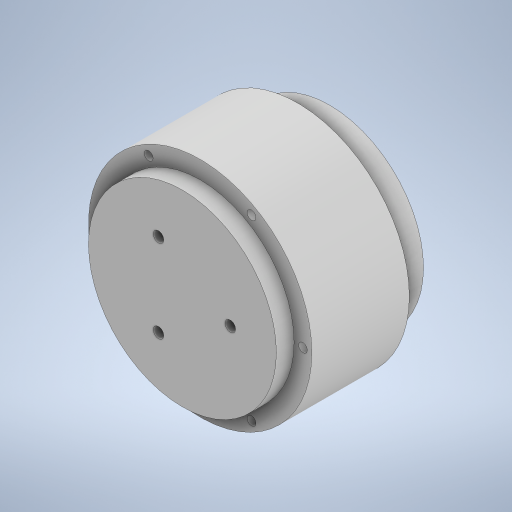
# Autodesk Inventor part: 부품1
Saved by Autodesk Inventor 2024 (Build 280153000, 153)
## iProperties
Created: 2024-03-08
Part Number: 부품1
Material: 일반
Document SubType Name: Modeling
Designer: unney
Density: 1 g/cm^3
Appearance: 기본값
Author: unney
Autodesk Inventor part; units mm, degrees
ref_plane "YZ Plane" through (0, 0, 0) normal (1, 0, 0) x (0, 1, 0)
ref_plane "XZ Plane" through (0, 0, 0) normal (0, 1, 0) x (-1, 0, 0)
ref_plane "XY Plane" through (0, 0, 0) normal (0, 0, 1) x (1, 0, 0)
sketch "스케치1" plane through (0, 0, 0) normal (0, 0, 1) x (1, 0, 0)
  circle A0 centre (0, 0) radius 31.5
  dimension "d0" = 63
  constraints: 1 centre point, 1 coincident
  measures "d0" diameter of A0
extrude "돌출1" add sketch "스케치1" along normal blind 27.5
sketch "스케치2" plane through (0, 0, 27.5) normal (0, 0, 1) x (1, 0, 0)
  circle A0 centre (0, 0) radius 26.5
  dimension "d3" = 53
  constraints: 1 centre point, 1 coincident
  measures "d3" diameter of A0
extrude "돌출2" add sketch "스케치2" along normal blind 5
sketch "스케치3" plane through (0, 0, 0) normal (0, 0, -1) x (-1, 0, 0)
  circle A0 centre (0, 0) radius 26.5 projected
  circle A1 centre (0, 0) radius 26.5
  dimension "d6" = 53
  constraints: 1 centre point, 1 coincident
  measures "d6" diameter of A1
extrude "돌출3" add sketch "스케치3" along normal blind 9
sketch "스케치5" plane through (0, 0, 32.5) normal (0, 0, 1) x (1, 0, 0)
  circle A0 centre (0, 0) radius 13.5
  circle A1 centre (-6.75, 11.6913) radius 1.5
  circle A2 centre (-6.75, -11.6913) radius 1.5
  circle A3 centre (13.5, 0) radius 1.5
  dimension "d19" = 360
  dimension "d39" = 360
  dimension "d13" = 27
  dimension "d43" = 360
  constraints: 4 centre point, 1 coincident, 9 other
  measures "d13" diameter of A0
extrude "돌출5" cut sketch "스케치5" against normal blind 3 contours A0 A3 | A0 A3 | A1 A0 | A0 A1 | A2 A0 | A0 A2
sketch "스케치6" plane through (0, 0, -9) normal (0, 0, -1) x (-1, 0, 0)
  circle A0 centre (0, 0) radius 24
  circle A1 centre (24, 0) radius 1.5
  circle A2 centre (12, 20.7846) radius 1.5
  circle A3 centre (-12, 20.7846) radius 1.5
  circle A4 centre (-24, 0) radius 1.5
  circle A5 centre (-12, -20.7846) radius 1.5
  circle A6 centre (12, -20.7846) radius 1.5
  dimension "d21" = 48
  dimension "d22" = 3
  dimension "d25" = 360
  constraints: 6 centre point, 1 coincident, 1 horizontal alignment, 15 other
  measures "d22" diameter of A1
extrude "돌출6" cut sketch "스케치6" against normal blind 8 contours A0 A1 | A0 A1 | A2 A0 | A0 A2 | A6 A0 | A0 A6 | A3 A0 | A0 A3 | A5 A0 | A0 A5 | A4 A0 | A0 A4
sketch "스케치7" plane through (0, 0, 0) normal (0, 0, -1) x (-1, 0, 0)
  circle A0 centre (0, 0) radius 29
  circle A1 centre (-29, 0) radius 1.25
  circle A2 centre (-14.5, -25.1147) radius 1.25
  circle A3 centre (14.5, -25.1147) radius 1.25
  circle A4 centre (29, 0) radius 1.25
  circle A5 centre (14.5, 25.1147) radius 1.25
  circle A6 centre (-14.5, 25.1147) radius 1.25
  dimension "d29" = 58
  dimension "d30" = 2.5
  dimension "d33" = 360
  constraints: 6 centre point, 1 coincident, 1 horizontal alignment, 15 other
  measures "d30" diameter of A1
extrude "돌출7" cut sketch "스케치7" against normal blind 53.25 contours A0 A4 | A0 A4 | A5 A0 | A0 A5 | A3 A0 | A0 A3 | A6 A0 | A0 A6 | A2 A0 | A0 A2 | A1 A0 | A0 A1
